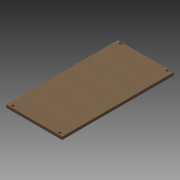
# Autodesk Inventor part: PS20001
Saved by Autodesk Inventor 2014 (Build 180170000, 170)
## iProperties
Category: NS
Created: 2013-07-16
Part Number: PS20001
Material: MDF Medium Density Fiberboard
Document SubType Name: Modeling
Designer: Edward
Density: 0.8 g/cm^3
Appearance: Cardboard - Corrugated
Description: MDF wasteboard (1/2")
Project: Shapeoko
Stock Number: PS20001
Vendor: A&M
User Status: W
Authority: PER A&M QOUOTE 8-7-13
Author: Edward
Subject: Structural
Comments: Fusion
Autodesk Inventor part; units mm, degrees
ref_plane "YZ Plane" through (0, 0, 0) normal (1, 0, 0) x (0, 1, 0)
ref_plane "XZ Plane" through (0, 0, 0) normal (0, 1, 0) x (-1, 0, 0)
ref_plane "XY Plane" through (0, 0, 0) normal (0, 0, 1) x (1, 0, 0)
sketch "Sketch1" plane through (0, 0, 0) normal (0, 0, 1) x (1, 0, 0)
  line L0 (-125, 250) -> (125, 250)
  line L1 (125, 250) -> (125, -250)
  line L2 (125, -250) -> (-125, -250)
  line L3 (-125, -250) -> (-125, 250)
  point P0 (0, 0)
  dimension "d0" = 250
  dimension "d1" = 500
  dimension "d2" = 125
  dimension "d3" = 250
  constraints: 8 end point, 2 parallel, 1 horizontal, 1 perpendicular
  measures "d0" distance of L1.end L2.end
  measures "d1" distance of L0.end L1.end
  measures "d2" distance from line of point (0, 0) L3
  measures "d3" distance from line of L0 point (0, 0)
extrude "Extrusion1" add sketch "Sketch1" along normal blind 12.7
sketch "Sketch2" plane through (0, 0, 12.7) normal (0, 0, 1) x (1, 0, 0)
  line L0 (-125, -250) -> (125, -250) projected
  line L1 (125, -250) -> (125, 250) projected
  circle A0 centre (105, -240) radius 2.75
  point P0 (0, 0)
  dimension "d6" = 5.5
  dimension "d7" = 10
  dimension "d8" = 20
  constraints: 1 centre point
  measures "d6" diameter of A0
  measures "d7" distance from line of L0 A0.centre
  measures "d8" distance from line of L1 A0.centre
hole "Hole1" at (105, -240, 12.7) direction (0, 0, -1) diameter 5.5 end through all counterbore diameter 11 counterbore depth 6
pattern_linear "Rectangular Pattern1" count 2 spacing 210 along (-1, 0, 0) count 2 spacing 480 along (0, 1, 0) of "Hole1"
sketch "Sketch4" plane through (0, 0, 12.7) normal (0, 0, 1) x (1, 0, 0)
  circle A0 centre (-105, 240) radius 5.5 projected
  circle A1 centre (105, 240) radius 5.5 projected
  line L0 (125, 250) -> (-125, 250) projected
  line L1 (-110.5, 240) -> (-110.5, 250)
  line L2 (-99.5, 240) -> (-99.5, 250)
  line L3 (99.5, 240) -> (99.5, 250)
  line L4 (110.5, 240) -> (110.5, 250)
  point P0 (0, 0)
  constraints: 8 end point, 4 point on circle, 4 point on line, 4 tangent, 3 perpendicular, 1 parallel
extrude "Extrusion2" cut sketch "Sketch4" against normal blind 6 contours A0 L1 L0 L2 | A1 L3 L0 L4
sketch "Sketch5" plane through (-105, 240, 6.7) normal (0, 0, 1) x (1, 0, 0)
  line L0 (-5.5, 10) -> (5.5, 10) projected
  circle A0 centre (0, 0) radius 2.75 projected
  arc A1 (204.5, 0) -> (215.5, 0) centre (210, 0) ccw projected
  line L1 (215.5, 10) -> (215.5, 0) projected
  line L2 (204.5, 10) -> (215.5, 10) projected
  line L3 (204.5, 0) -> (204.5, 10) projected
  circle A2 centre (210, 0) radius 2.75 projected
  line L4 (-2.75, 0) -> (-2.75, 10)
  line L5 (2.75, 0) -> (2.75, 10)
  line L6 (212.75, 0) -> (212.75, 10)
  line L7 (207.25, 0) -> (207.25, 10)
  point P0 (105, -240)
  constraints: 8 end point, 4 point on circle, 4 point on line, 4 tangent, 3 perpendicular, 1 parallel
extrude "Extrusion3" cut sketch "Sketch5" against normal through all contours L0 L5 A0 L4 | L2 L6 A2 L7
equation "\"d2\" = 0.5 * d0"
equation "\"d3\" = 0.5 * d1"
body "Solid1"
